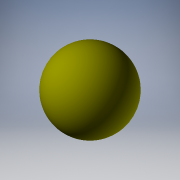
# Autodesk Inventor part: SKF_W 61810-2RS1_PART3
Saved by Autodesk Inventor 2019 (Build 230136000, 136)
## iProperties
Created: 2022-09-01
Part Number: SKF_W 61810-2RS1_PART3
Material: Generic
Catalog Web Link: www.cadenas.de
Description: -Deep groove ball bearings
Vendor: SKF
Document SubType Name: Modeling
Designer: psAdmin
Manufacturer: SKF
Mass: 51 g
Surface Area: 0.494894 cm^2
Volume: 0.0327372 cm^3
Density: 1 g/cm^3
Appearance: PSOLRGB-192-192-192
Category: PARTsolutions
Company: SKF
Title: SKF_W 61810-2RS1_PART3
Author: Cadenas PARTsolutions
Comments: Deep groove ball bearings
PSOL_IDENT_0: {$CADENAS_DATA/23d-libs/skf/bearings_units_and_housings/ball_bearings/deep_groove_ball_bearings/bb1_
PSOL_IDENT_1: 001_101.prj},211 {VTYP=3D},{NB=SKF_W 61810-2RS1_PART3},{LINA=SKF_W 61810-2RS1_PART3},{NN=BB1_001_101
PSOL_IDENT_2: _PART3},{NOPRJ=TRUE},{DATE=04.08.2022 15:25:15},{GEOMDATE=04.07.2022 10:54:51},{VERSION=},{LINEID=19
PSOL_IDENT_3: 000},{WBVAR=},{WBNUMERIC=}  {NB=SKF_W 61810-2RS1_PART3},{LINA=SKF_W 61810-2RS1_PART3},{KT=DUMMY},{DE
PSOL_IDENT_4: SIGNATION=W 61810-2RS1},{R12=0.30},{DD=50.000},{D=65.000},{B=7.000},{C=},{CX=},{CXX=},{CA=0.000},{XX
PSOL_IDENT_5: VARIANT=},{XXDESIGN=Single row stainless steel},{XXSEALING=Contact seal on both sides},{DESIGN=dgbbw
PSOL_IDENT_6: 2rs},{DESIGNIR=dgbbw2rs},{VARIANT=},{DD1=54.67},{DD2=54.67},{DD2X=},{DD2A=54.67},{D1=60.30},{D1X=0.0
PSOL_IDENT_7: 0},{D2=61.55},{D2A=61.55},{D3=},{D3X=},{D3A=0.000},{D4=},{HH=0.000},{BB=0.000},{BBX=},{BBA=0.000},{F
PSOL_IDENT_8: F=},{R0MAX=0.000},{R0=0.000},{PITCH=57.50},{DW=3.969},{DDAMIN=52.000},{DDAMAX=54.500},{DDBMIN=0.000}
PSOL_IDENT_9: ,{DDBMAX=0.000},{DBMIN=0.000},{DAMAX=63.000},{BBAMIN=0.000},{CAMAX=0.000},{RAMAX=0.300},{LOAD1=5.070
PSOL_IDENT_10: },{LOAD2=5.500},{LOAD3=0.236},{SPEED1=0},{SPEED2=6000},{KR=0.020},{F0=15.300},{Z=23},{II=1},{MASS=0.
PSOL_IDENT_11: 051},{BEARING=W 61810-2RS1},{RING=},{HELP=2.350},{HELP2=1.725},{DD1ALG=27.335},{YALG=27.335},{PITCH1=
PSOL_IDENT_12: 57.500},{DW1=3.969},{YALG1=30.150},{HALG1=2.350},{SH=27.335},{CU=0.606},{HALG=2.335},{B1=0},{SHIELDH
PSOL_IDENT_13: ELP=2},{D4A=0.000},{FFA=0.000},{RS1=},{HELP3=0}
NB: SKF_W 61810-2RS1_PART3
NT: Deep groove ball bearings
NBSYN: SKF_$DESIGNATION._PART3
LINA: SKF_W 61810-2RS1_PART3
CATALOG: SKF
DESIGNATION: W 61810-2RS1
R12: 0.3
DD: 50
D: 65
B: 7
XXDESIGN: Single row stainless steel
XXSEALING: Contact seal on both sides
DD2: 54.67
D2: 61.55
LOAD1: 5.07
LOAD2: 5.5
LOAD3: 0.236
SPEED1: 0
SPEED2: 6000
BEARING: W 61810-2RS1
SUPPLIER: SKF
ARTICLENO: SKF_W 61810-2RS1_PART3
BOMINFO: SKF_W 61810-2RS1_PART3
CREATOR: CADENAS GmbH
Autodesk Inventor part; units mm, degrees
ref_plane "YZ Plane" through (0, 0, 0) normal (1, 0, 0) x (0, 1, 0)
ref_plane "XZ Plane" through (0, 0, 0) normal (0, 1, 0) x (-1, 0, 0)
ref_plane "XY Plane" through (0, 0, 0) normal (0, 0, 1) x (1, 0, 0)
sketch "Sketch_6" plane through (0, 0, 0) normal (0, 0, 1) x (1, 0, 0)
  line L0 (5.4845, 28.75) -> (1.5155, 28.75)
  arc A0 (5.4845, 28.75) -> (1.5155, 28.75) centre (3.5, 28.75) ccw
  line L1 (5.4845, 28.75) -> (1.5155, 28.75)
  dimension "d0" = 360
  constraints: 4 end point, 2 point on circle, 1 centre point
revolve "Revolution1" add sketch "Sketch_6" angle 360 about axis through (5.4845, 28.75, 0) along (1, 0, 0)
body "Solid1"
